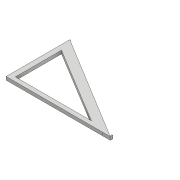
# Autodesk Inventor part: Part2
Saved by Autodesk Inventor 2017 (Build 210142000, 142)
## iProperties
Created: 2019-07-20
Part Number: Part2
Material: Generic
Document SubType Name: Modeling
Designer: Admin
Density: 1 g/cm^3
Appearance: Default
Author: Admin
Autodesk Inventor part; units mm, degrees
ref_plane "YZ Plane" through (0, 0, 0) normal (1, 0, 0) x (0, 1, 0)
ref_plane "XZ Plane" through (0, 0, 0) normal (0, 1, 0) x (-1, 0, 0)
ref_plane "XY Plane" through (0, 0, 0) normal (0, 0, 1) x (1, 0, 0)
sketch "Sketch1" plane through (0, 0, 0) normal (0, 0, 1) x (1, 0, 0)
  line L0 (0, 0) -> (0, 365)
  line L1 (0, 365) -> (597.3065, 0)
  line L2 (597.3065, 0) -> (0, 0)
  dimension "d0" = 365
  dimension "d1" = 700
  constraints: 6 end point, 1 perpendicular, 1 vertical
  measures "d0" distance of L0.start L0.end
  measures "d1" distance of L0.end L1.end
extrude "Extrusion1" add sketch "Sketch1" along normal blind 20
sketch "Sketch2" plane through (0, 0, 20) normal (0, 0, 1) x (1, 0, 0)
  line L0 (30.8422, 26.0696) -> (30.8422, 311.5961)
  line L1 (0, 365) -> (0, 0) projected
  line L2 (30.8422, 311.5961) -> (501.2951, 26.0696)
  line L3 (501.2951, 26.0696) -> (30.8422, 26.0696)
  constraints: 6 end point, 1 parallel, 1 perpendicular
extrude "Extrusion2" cut sketch "Sketch2" against normal blind 161.75
sketch "Sketch3" plane through (0, 0, 20) normal (0, 0, 1) x (1, 0, 0)
  line L0 (0, 365) -> (597.3065, 0) projected
  line L1 (0, 365) -> (0, 393.2795)
  line L2 (0, 393.2795) -> (643.5846, 0)
  line L3 (597.3065, 0) -> (643.5846, 0)
  point P0 (0, 0)
  constraints: 6 end point, 1 horizontal, 1 parallel, 1 vertical
extrude "Extrusion3" add sketch "Sketch3" against normal blind 4
sketch "Sketch4" plane through (0, 0, 0) normal (0, 0, -1) x (-1, 0, 0)
  line L0 (-597.3065, 0) -> (0, 0) projected
  line L1 (-643.5846, 0) -> (-597.3065, 0) projected
  line L2 (-597.3065, 0) -> (-643.5846, 0)
  line L3 (0, 365) -> (0, 393.2795) projected
  line L4 (-643.5846, 0) -> (0, 393.2795)
  line L5 (0, 393.2795) -> (0, 365)
  line L6 (0, 365) -> (-597.3065, 0)
  constraints: 8 end point, 2 collinear, 1 parallel
extrude "Extrusion4" add sketch "Sketch4" against normal blind 4
sketch "Sketch5" plane through (0, 0, 0) normal (0, -1, 0) x (1, 0, 0)
  line L0 (597.3065, 4) -> (643.5846, 4) projected
  line L1 (643.5846, 20) -> (643.5846, 16) projected
  line L2 (643.5846, 4) -> (643.5846, 16)
  line L3 (597.3065, 4) -> (597.3065, 16) projected
  line L4 (643.5846, 16) -> (597.3065, 16)
  line L5 (597.3065, 16) -> (597.3065, 4)
  point P0 (0, 0)
  constraints: 6 end point, 1 collinear, 1 perpendicular, 1 vertical
extrude "Extrusion5" add sketch "Sketch5" against normal blind 2.75
sketch "Sketch6" plane through (643.5846, 0, 16) normal (1, 0, 0) x (0, 0, -1)
  line L0 (-4, 0) -> (-4, 393.2795) projected
  line L1 (16, 0) -> (-4, 0)
  line L2 (-4, 0) -> (-4, 15)
  line L3 (-4, 15) -> (16, 15)
  line L4 (16, 15) -> (16, 0)
  dimension "d12" = 15
  constraints: 8 end point, 2 parallel, 1 horizontal, 1 perpendicular, 1 point on line
  measures "d12" distance of L1.end L2.end
extrude "Extrusion6" add sketch "Sketch6" against normal blind 5
sketch "Sketch7" plane through (0, 0, 0) normal (-1, 0, 0) x (0, 0, 1)
  line L0 (0, 0) -> (0, 393.2795) projected
  line L1 (20, 3.0554) -> (20, 393.2795) projected
  line L2 (0, 393.2795) -> (20, 393.2795)
  line L3 (20, 393.2795) -> (20, 363.4031)
  line L4 (20, 363.4031) -> (0, 363.4031)
  line L5 (0, 363.4031) -> (0, 393.2795)
  constraints: 8 end point, 2 parallel, 1 horizontal, 1 perpendicular, 1 point on line
extrude "Extrusion7" add sketch "Sketch7" against normal blind 5
body "Solid1"
